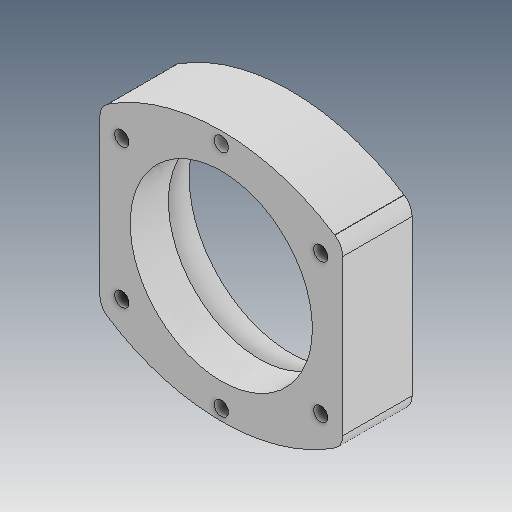
# Autodesk Inventor part: Tilting head - extended part
Saved by Autodesk Inventor 2020.3 (Build 243373010, 373A)
## iProperties
Created: 2021-05-11
Part Number: Tilting head - extended part
Material: Steel, Carbon
Document SubType Name: Modeling
Designer: marti
Density: 7.85 g/cm^3
Appearance: Semi-Polished
Author: marti
Autodesk Inventor part; units mm, degrees
ref_plane "YZ Plane" through (0, 0, 0) normal (1, 0, 0) x (0, 1, 0)
ref_plane "XZ Plane" through (0, 0, 0) normal (0, 1, 0) x (-1, 0, 0)
ref_plane "XY Plane" through (0, 0, 0) normal (0, 0, 1) x (1, 0, 0)
sketch "Sketch1" plane through (0, 0, 0) normal (0, 0, 1) x (1, 0, 0)
  circle A0 centre (28.6703, -20.0752) radius 2.067
  circle A1 centre (-28.6703, 20.0752) radius 2.067
  circle A2 centre (-28.6703, -20.0752) radius 2.067
  circle A3 centre (28.6703, 20.0752) radius 2.067
  circle A4 centre (0, 33) radius 2.067
  circle A5 centre (0, -33) radius 2.067
  spline S0 degree 3 poles (-33.0232, -26.3606) (-33.4707, -26.0209) (-33.8582, -25.6078) (-34.4385, -24.7312) (-34.6469, -24.2869) (-34.9285, -23.3518) (-35, -22.866) (-35, -22.3776) knots 0.026434 0.026434 0.026434 0.026434 0.19535 0.19535 0.341801 0.341801 0.488319 0.488319 0.488319 0.488319
  arc A6 (-33.0232, -26.3606) -> (33.0232, -26.3606) centre (0, 23.734) ccw
  spline S1 degree 3 poles (35, -22.3776) (35, -23.0287) (34.8729, -23.6735) (34.4404, -24.7277) (34.1898, -25.15) (33.6298, -25.8399) (33.3414, -26.119) (33.0232, -26.3606) knots 0 0 0 0 0.195306 0.195306 0.341836 0.341836 0.461894 0.461894 0.461894 0.461894
  line L0 (35, -22.3776) -> (35, 22.3638)
  spline S2 degree 3 poles (32.722, 26.5579) (33.2681, 26.2035) (33.7398, 25.7458) (34.3984, 24.7948) (34.6216, 24.3377) (34.9233, 23.3723) (35, 22.8695) (35, 22.3638) knots 0 0 0 0 0.195321 0.195321 0.347039 0.347039 0.498754 0.498754 0.498754 0.498754
  spline S3 degree 3 poles (32.6565, 26.6005) (32.6783, 26.5863) (32.7001, 26.5721) (32.722, 26.5579) knots 0 0 0 0 0.007808 0.007808 0.007808 0.007808
  arc A7 (32.6565, 26.6005) -> (-32.6565, 26.6005) centre (0, -23.734) ccw
  spline S4 degree 3 poles (-32.6565, 26.6005) (-32.6783, 26.5863) (-32.7001, 26.5721) (-32.722, 26.5579) knots -3.47 -3.47 -3.47 -3.47 -3.462013 -3.462013 -3.462013 -3.462013
  spline S5 degree 3 poles (-35, 22.3638) (-35, 23.0149) (-34.8728, 23.6598) (-34.4336, 24.7299) (-34.1718, 25.166) (-33.5262, 25.9446) (-33.1462, 26.2826) (-32.722, 26.5579) knots 0 0 0 0 0.195326 0.195326 0.347039 0.347039 0.498754 0.498754 0.498754 0.498754
  line L1 (-35, 22.3638) -> (-35, -22.3776)
  circle A8 centre (0, 0) radius 26.25
  dimension "d2" = 33
  dimension "d3" = 33
  constraints: 9 centre point, 4 end point, 4 point on circle, 18 other
  measures "d2" distance of point (0, 0) A4.centre
  measures "d3" distance of A5.centre point (0, 0)
extrude "Extrusion1" add sketch "Sketch1" along normal blind 20
sketch "Sketch2" plane through (0, 0, 0) normal (0, 0, -1) x (-1, 0, 0)
  circle A0 centre (0, 0) radius 29.2625
  dimension "d4" = 58.525
  constraints: 1 centre point, 1 coincident
  measures "d4" diameter of A0
extrude "Extrusion2" cut sketch "Sketch2" against normal blind 9
body "Solid1"
